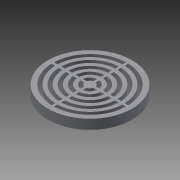
# Autodesk Inventor part: Lattice 2
Saved by Autodesk Inventor 2013 (Build 170138000, 138)
## iProperties
Created: 2014-07-03
Part Number: Lattice 2
Material: Genérico
Document SubType Name: Chapa
Designer: Administrador
Density: 1 g/cm^3
Sheet Metal Rule: Por defecto_mm
Author: Administrador
Autodesk Inventor part; units mm, degrees
ref_plane "YZ Plane" through (0, 0, 0) normal (1, 0, 0) x (0, 1, 0)
ref_plane "XZ Plane" through (0, 0, 0) normal (0, 1, 0) x (-1, 0, 0)
ref_plane "XY Plane" through (0, 0, 0) normal (0, 0, 1) x (1, 0, 0)
sketch "Boceto1" plane through (0, 0, 0) normal (0, 0, 1) x (1, 0, 0)
  circle A0 centre (0, 0) radius 17.5
  circle A1 centre (0, 0) radius 15.5
  dimension "d0" = 35
  dimension "d1" = 31
  constraints: 2 centre point
  measures "d0" diameter of A0
  measures "d1" diameter of A1
extrude "Extrusión1" add sketch "Boceto1" along normal blind 2
sketch "Boceto2" plane through (0, 0, 2) normal (0, 0, 1) x (1, 0, 0)
  circle A0 centre (0, 0) radius 17.5 projected
extrude "Extrusión2" add sketch "Boceto2" along normal blind 2
sketch "Boceto3" plane through (0, 0, 2) normal (0, 0, -1) x (-1, 0, 0)
  circle A0 centre (0, 0) radius 15.5 projected
  circle A1 centre (0, 0) radius 15.5 projected
  circle A2 centre (0, 0) radius 14
  circle A3 centre (0, 0) radius 12.5
  circle A4 centre (0, 0) radius 11
  circle A5 centre (0, 0) radius 9.5
  circle A6 centre (0, 0) radius 8
  circle A7 centre (0, 0) radius 6.5
  circle A8 centre (0, 0) radius 5
  circle A9 centre (0, 0) radius 3.5
  circle A10 centre (0, 0) radius 2
  line L0 (-0.5014, 1.9361) -> (-0.5014, 2)
  line L1 (-0.5014, 1.9361) -> (-0.5014, 15.5)
  line L2 (-0.5014, 1.9361) -> (13.0625, 1.9361) construction
  line L3 (0.5019, 1.9361) -> (0.5019, 15.5)
  line L4 (0.5019, 1.9361) -> (0.5019, -15.5)
  line L5 (-0.5014, 1.9361) -> (-0.5014, -15.5)
  line L6 (1.9361, 0.5016) -> (15.5, 0.5016)
  line L7 (1.9361, -0.5011) -> (15.5, -0.5011)
  line L8 (1.9361, -0.5011) -> (-15.5, -0.5011)
  line L9 (1.9361, 0.5016) -> (-15.5, 0.5016)
  dimension "d7" = 28
  dimension "d8" = 25
  dimension "d9" = 22
  dimension "d10" = 19
  dimension "d11" = 16
  dimension "d12" = 13
  dimension "d13" = 10
  dimension "d14" = 7
  dimension "d15" = 4
  dimension "d16" = 90
  constraints: 20 end point, 9 centre point, 1 horizontal, 1 perpendicular
  measures "d7" diameter of A2
  measures "d8" diameter of A3
  measures "d9" diameter of A4
  measures "d10" diameter of A5
  measures "d11" diameter of A6
  measures "d12" diameter of A7
  measures "d13" diameter of A8
  measures "d14" diameter of A9
  measures "d15" diameter of A10
  measures "d16" angle of L2 L1
extrude "Extrusión3" cut sketch "Boceto3" against normal blind 2 contours A0 L7 A2 L6 | L6 A2 L3 A0 | A0 L4 A2 L7 | L3 A2 L1 A0 | A0 L5 A2 L4 | L1 A2 L9 A0 | L6 A4 L3 A3 | A3 L7 A4 L6 | A0 L8 A2 L5 | A3 L4 A4 L7 | L9 A2 L8 A0 | L3 A4 L1 A3 | A3 L5 A4 L4 | L1 A4 L9 A3 | L6 A6 L3 A5 | A5 L7 A6 L6 | A3 L8 A4 L5 | A5 L4 A6 L7 | L9 A4 L8 A3 | L3 A6 L1 A5 | A5 L5 A6 L4 | L1 A6 L9 A5 | L6 A8 L3 A7 | A7 L7 A8 L6 | A5 L8 A6 L5 | A7 L4 A8 L7 | L9 A6 L8 A5 | L3 A8 L1 A7 | A7 L5 A8 L4 | L1 A8 L9 A7 | L6 A10 L3 A9 | A9 L7 A10 L6 | A7 L8 A8 L5 | A9 L4 A10 L7 | L9 A8 L8 A7 | L3 A10 L0 L1 A9 | A9 L5 A10 L4 | L1 L0 A10 L9 A9 | A9 L8 A10 L5 | L9 A10 L8 A9
sketch "Boceto4" plane through (0, 0, 4) normal (0, 0, 1) x (1, 0, 0)
  line L0 (-16.1458, 0.5) -> (16.1458, 0.5)
  line L1 (16.1458, 0.5) -> (16.1458, -0.5)
  line L2 (16.1458, -0.5) -> (-16.1458, -0.5)
  line L3 (-16.1458, -0.5) -> (-16.1458, 0.5)
  line L4 (-16.1458, 0.5) -> (16.1458, -0.5) construction
  line L5 (16.1458, 0.5) -> (-16.1458, -0.5) construction
  line L6 (-0.5, -16.1458) -> (0.5, -16.1458)
  line L7 (0.5, -16.1458) -> (0.5, 16.1458)
  line L8 (0.5, 16.1458) -> (-0.5, 16.1458)
  line L9 (-0.5, 16.1458) -> (-0.5, -16.1458)
  line L10 (-0.5, -16.1458) -> (0.5, 16.1458) construction
  line L11 (0.5, -16.1458) -> (-0.5, 16.1458) construction
  point P0 (0, 0)
  point P1 (0, 0)
  dimension "d19" = 1
  dimension "d20" = 1
  constraints: 24 end point, 4 midpoint, 4 parallel, 2 horizontal, 2 perpendicular
  measures "d19" distance of L0.end L1.end
  measures "d20" distance of L8.end L7.end
extrude "Extrusión4" add sketch "Boceto4" against normal blind 2
equation "\"Radio_pliegue\" = Grosor"
equation "\"Anchura_desahogo_plegado\" = Grosor"
equation "\"Profundidad_desahogo_plegado\" = 0.5 * Grosor"
equation "\"Tamaño_destalonado\" = 4 * Grosor"
equation "\"Remanente_mínimo\" = 2 * Grosor"
equation "\"Radiodetransición\" = Radio_pliegue"
equation "\"Tamaño_de_radio_de_Jacobi\" = Radio_pliegue"
equation "\"TamañoSeparación\" = Grosor"
equation "\"Grosor\" = 0.5"
